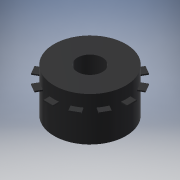
# Autodesk Inventor part: ExtruderCouplingBowden
Saved by Autodesk Inventor 2016 (Build 200138000, 138)
## iProperties
Category: Hardware
Created: 2015-10-25
Part Number: ExtruderCouplingBowden
Material: ABS Plastic
Document SubType Name: Modeling
Designer: Jack
Density: 1.06 g/cm^3
Appearance: Smooth - Dark Gray
Vendor: E3D
Author: Jack
Title: Embedded Bowden Coupling 1.75
Autodesk Inventor part; units mm, degrees
ref_plane "YZ Plane" through (0, 0, 0) normal (1, 0, 0) x (0, 1, 0)
ref_plane "XZ Plane" through (0, 0, 0) normal (0, 1, 0) x (-1, 0, 0)
sketch "Sketch1" plane through (0, 0, 0) normal (0, 0, 1) x (1, 0, 0)
  circle A0 centre (0, 0) radius 5.75
  dimension "d0" = 11.5
  constraints: 1 centre point, 1 coincident
  measures "d0" diameter of A0
extrude "Extrusion1" add sketch "Sketch1" along normal blind 7
ref_plane "Work Plane1" through (0, 0, 5) normal (0, 0, 1) x (1, 0, 0)
sketch "Sketch2" plane through (0, 0, 5) normal (0, 0, 1) x (1, 0, 0)
  circle A0 centre (0, 0) radius 5.75 projected
  circle A1 centre (0, 0) radius 5.75 projected
  line L0 (-0.75, 5.7009) -> (-0.75, 6.7009)
  line L1 (-0.75, 6.7009) -> (0.75, 6.7009)
  line L2 (0.75, 6.7009) -> (0.75, 5.7009)
  dimension "d4" = 1.5
  dimension "d5" = 1
  constraints: 6 end point, 4 point on circle, 2 vertical, 1 parallel, 1 perpendicular
  measures "d4" distance of L0.end L1.end
  measures "d5" distance of L1.end L2.end
extrude "Extrusion2" add sketch "Sketch2" along normal mid plane 0.2 contours A0 L0 L1 L2
pattern_circular "Circular Pattern1" count 12 over 360 about axis through (0, 0, 0) along (0, 0, 1) of "Extrusion2"
sketch "Sketch3" plane through (0, 0, 7) normal (0, 0, 1) x (1, 0, 0)
  circle A0 centre (0, 0) radius 5.75 projected
hole "Hole1" at (0, 0, 7) direction (0, 0, -1) diameter 4 end through all
body "Solid1"
